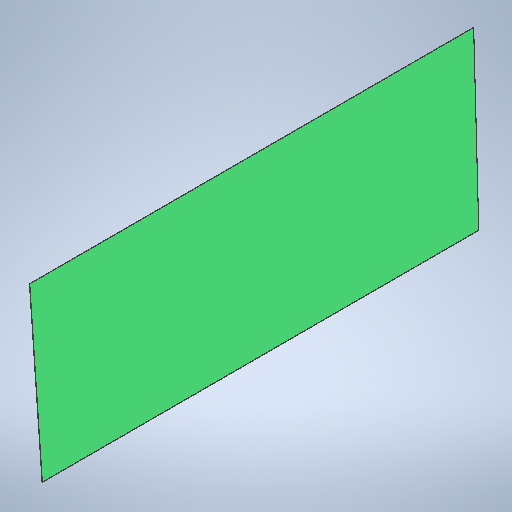
# Autodesk Inventor part: GBK dummy wall 4
Saved by Autodesk Inventor 2026.2 (Build 302298000, 298)
## iProperties
Created: 2026-05-13
Part Number: GBK dummy wall 4
Material: Generic
Document SubType Name: Modeling
Designer: admin
Density: 1 g/cm^3
Appearance: Default
Author: admin
Autodesk Inventor part; units mm, degrees
ref_plane "YZ Plane" through (0, 0, 0) normal (1, 0, 0) x (0, 1, 0)
ref_plane "XZ Plane" through (0, 0, 0) normal (0, 1, 0) x (-1, 0, 0)
ref_plane "XY Plane" through (0, 0, 0) normal (0, 0, 1) x (1, 0, 0)
sketch "Sketch1" plane through (0, 0, 0) normal (0, 0, 1) x (1, 0, 0)
  line L0 (355.835, 0) -> (345.835, 0)
  line L1 (345.835, 0) -> (110.0274, 4499.4774)
  line L2 (110.0274, 4499.4774) -> (120, 4500)
  line L3 (120, 4500) -> (355.835, 0)
  line L4 (0, 4500) -> (0, 0)
  dimension "d0" = 10
  dimension "d1" = 87
  dimension "d2" = 4500
  dimension "d5" = 120
  constraints: 10 end point, 2 perpendicular, 1 horizontal, 1 horizontal alignment, 1 point on line, 1 vertical
  measures "d0" distance of L0.start L0.end
  measures "d1" angle of L0 L1
  measures "d2" distance from line of L0 L2.end
  measures "d5" distance of L2.end L4.start
extrude "Extrusion1" add sketch "Sketch1" against normal blind 12000
sketch "Sketch2" plane through (0, 0, 0) normal (1, 0, 0) x (0, 1, 0)
  line L0 (0, 0) -> (4500, 0) projected
  line L1 (0, 0) -> (0, -12000) projected
  line L2 (4500, -12000) -> (0, -12000) projected
  line L3 (4500, 0) -> (4500, -12000) projected
  line L4 (4500, -100) -> (0, -200)
  line L5 (4500, -11900) -> (0, -11800)
  line L6 (4500, -6000) -> (0, -6000) construction
  dimension "d6" = 100
  dimension "d10" = 200
  constraints: 6 end point, 4 point on line, 2 midpoint, 1 other
  measures "d6" distance of L2.start L5.start
  measures "d10" distance of L5.end L1.end
extrude "Extrusion2" cut sketch "Sketch2" along normal through all contours L0 L3 L4 L1 | L5 L3 L2 L1
body "Solid1"
